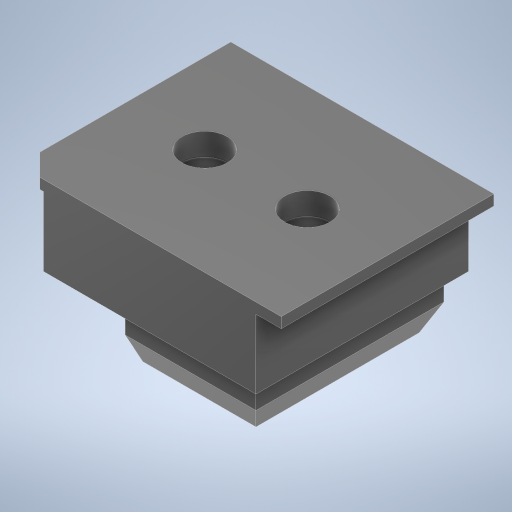
# Autodesk Inventor part: Header Larger Area
Saved by Autodesk Inventor 2024 (Build 280153000, 153)
## iProperties
Created: 2023-11-07
Part Number: Header Larger Area
Material: Acetal Resin, Black
Document SubType Name: Modeling
Designer: jamha
Density: 1.425 g/cm^3
Appearance: Smooth - Black
Author: jamha
Autodesk Inventor part; units mm, degrees
ref_plane "YZ Plane" through (0, 0, 0) normal (1, 0, 0) x (0, 1, 0)
ref_plane "XZ Plane" through (0, 0, 0) normal (0, 1, 0) x (-1, 0, 0)
ref_plane "XY Plane" through (0, 0, 0) normal (0, 0, 1) x (1, 0, 0)
ref_plane "Work Plane2" through (0, 3.81, 0) normal (0, 1, 0) x (1, 0, 0)
sketch "Sketch2" plane through (0, 3.81, 0) normal (0, 1, 0) x (1, 0, 0)
  line L0 (-29.21, 29.21) -> (1.27, 29.21)
  line L1 (1.27, -1.27) -> (-29.21, -1.27)
  line L2 (-29.21, -1.27) -> (-29.21, 29.21)
  line L3 (1.27, -1.27) -> (1.27, 29.21)
  line L4 (-4.8761, 25.94) -> (-25.94, 25.94) projected
  line L5 (-25.94, 25.94) -> (-25.94, 0) projected
  line L6 (-25.94, 0) -> (0, 0) projected
  line L7 (0, 0) -> (0, 21.0639) projected
  dimension "d3" = 30.48
  constraints: 8 end point, 3 equal length, 1 horizontal, 1 parallel, 1 vertical
  measures "d3" distance of L1.end L0.start
extrude "Extrusion2" add sketch "Sketch2" along normal blind 11.43
ref_plane "Work Plane1" through (0, -3.81, 0) normal (0, -1, 0) x (1, 0, 0)
ref_plane "Work Plane4" through (1.27, 3.81, -29.21) normal (0, 0, -1) x (-1, 0, 0)
sketch "Sketch6" plane through (1.27, 3.81, -29.21) normal (0, 0, -1) x (-1, 0, 0)
  line L0 (0, 11.43) -> (30.48, 11.43) projected
  line L1 (0, 11.43) -> (-7.239, 11.43)
  line L2 (-7.239, 11.43) -> (-7.239, 9.9183)
  line L3 (-7.239, 9.9183) -> (0, 9.9183)
  line L4 (0, 9.9183) -> (0, 11.43)
  line L5 (15.24, 11.43) -> (15.24, -7.62) construction
  line L6 (1.27, -7.62) -> (27.21, -7.62) construction
  line L7 (30.48, 11.43) -> (37.719, 11.43)
  line L8 (37.719, 11.43) -> (37.719, 9.9183)
  line L9 (37.719, 9.9183) -> (30.48, 9.9183)
  line L10 (30.48, 9.9183) -> (30.48, 11.43)
  point P0 (1.27, -3.81)
  dimension "d22" = 7.239
  constraints: 18 end point, 3 symmetric about line, 2 parallel, 1 horizontal, 1 midpoint, 1 perpendicular, 1 vertical, 2 other
  measures "d22" distance of L2.end L3.end
extrude "Extrusion6" add sketch "Sketch6" against normal up to surface (30.48 mm away)
ref_plane "Work Plane3" through (0, 15.24, 0) normal (0, 1, 0) x (1, 0, 0)
sketch "Sketch9" plane through (0, 15.24, 0) normal (0, 1, 0) x (1, 0, 0)
  line L0 (8.509, 29.21) -> (8.509, -1.27) construction
  line L1 (8.509, 13.97) -> (-36.449, 13.97) construction
  line L2 (-36.449, 29.21) -> (-36.449, -1.27) construction
  line L3 (-36.449, -1.27) -> (8.509, -1.27) construction
  line L4 (-13.97, -1.27) -> (-13.97, 29.21) construction
  line L5 (-36.449, 29.21) -> (8.509, 29.21) construction
  circle A0 centre (-21.336, 13.97) radius 3.2512
  circle A1 centre (-6.604, 13.97) radius 3.2512
  line L6 (-6.604, 13.97) -> (-21.336, 13.97) construction
  point P0 (0, 0)
  point P1 (-13.97, 13.97)
  point P2 (-13.97, 13.97)
  point P3 (-13.97, 13.97)
  point P4 (-13.97, 13.97)
  dimension "d25" = 14.732
  constraints: 6 end point, 6 midpoint, 3 coincident, 2 centre point, 1 horizontal
  measures "d25" distance of L6.end L6.start
extrude "Extrusion8" cut sketch "Sketch9" against normal blind 3.2258
ref_plane "Work Plane5" through (0, 15.24, 0) normal (0, 1, 0) x (1, 0, 0)
sketch "Sketch10" plane through (0, 15.24, 0) normal (0, 1, 0) x (1, 0, 0)
  line L0 (-29.21, -1.27) -> (-29.21, 29.21) projected
  line L1 (1.27, 29.21) -> (1.27, -1.27) projected
  line L2 (-36.449, 29.21) -> (-36.449, -1.27) projected
  line L3 (-36.449, 29.21) -> (8.509, 29.21) projected
  line L4 (-36.449, -1.27) -> (8.509, -1.27) projected
  line L5 (8.509, 29.21) -> (8.509, -1.27) projected
  line L6 (-29.21, 29.21) -> (-36.449, 29.21) projected
  line L7 (-29.21, 29.21) -> (-36.449, 29.21)
  line L8 (-32.8295, 29.21) -> (-32.8295, -1.27)
  line L9 (8.509, 29.21) -> (1.27, 29.21)
  line L10 (4.8895, 29.21) -> (4.8895, -1.27)
  line L11 (8.509, -1.27) -> (4.8895, -1.27)
  line L12 (8.509, 29.21) -> (8.509, -1.27) projected
  line L13 (8.509, 29.21) -> (8.509, -1.27)
  point P0 (0, 0)
  constraints: 12 end point, 4 collinear, 2 midpoint, 2 perpendicular, 2 point on line
extrude "Extrusion9" cut sketch "Sketch10" against normal blind 25.4 contours L4 L2 L3 L8 | L10 L3 L5 L4
sketch "Sketch18" plane through (0, 3.81, 0) normal (0, -1, 0) x (1, 0, 0)
  line L0 (1.27, 1.27) -> (1.27, -29.21) construction
  line L1 (1.27, -13.97) -> (-29.21, -13.97) construction
  line L2 (-29.21, -29.21) -> (-29.21, 1.27) construction
  line L3 (1.27, -29.21) -> (-29.21, -29.21) construction
  line L4 (-13.97, -29.21) -> (-13.97, 0) construction
  line L5 (0, -13.97) -> (-27.94, -13.97) construction
  line L6 (-13.97, 0) -> (-13.97, -27.94) construction
  line L7 (-13.97, -27.94) -> (-35.862, -27.94) construction
  line L8 (-20.7022, -26.44) -> (-37.4547, -26.44) construction
  line L9 (-27.44, -0.5) -> (-0.5, -0.5)
  line L10 (-0.5, -0.5) -> (-0.5, -27.44)
  line L11 (-0.5, -27.44) -> (-27.44, -27.44)
  line L12 (-27.44, -27.44) -> (-27.44, -0.5)
  line L13 (-27.44, -0.5) -> (-0.5, -27.44) construction
  line L14 (-0.5, -0.5) -> (-27.44, -27.44) construction
  line L15 (-27.44, -8.9624) -> (-18.9776, -0.5)
  point P0 (-13.97, -13.97)
  point P1 (-27.44, -20.8093)
  point P2 (-20.3093, -27.44)
  dimension "d66" = 1.27
  dimension "d72" = 26.94
  constraints: 26 end point, 7 midpoint, 5 point on line, 4 perpendicular, 2 horizontal, 2 parallel, 1 vertical
  measures "d66" distance between parallel lines of L3 L7
  measures "d72" distance of L10.end L11.end
extrude "Extrusion15" add sketch "Sketch18" along normal blind 7.62
sketch "Sketch19" plane through (0, -3.81, 0) normal (0, -1, 0) x (1, 0, 0)
  line L0 (-2.278, -2.278) -> (-2.278, -25.662) construction
  line L1 (-2.278, -13.97) -> (-25.662, -13.97) construction
  line L2 (-25.662, -25.662) -> (-25.662, -2.278) construction
  line L3 (-25.662, -2.278) -> (-2.278, -2.278) construction
  line L4 (-13.97, -2.278) -> (-13.97, -25.15) construction
  circle A0 centre (-13.97, -13.714) radius 2.0193
  point P0 (0, 0)
  point P1 (-25.412, -19.8229)
  dimension "d79" = 4.0386
  constraints: 4 end point, 3 midpoint, 1 centre point, 1 horizontal, 1 vertical, 2 other
  measures "d79" diameter of A0
extrude "Extrusion16" cut sketch "Sketch19" against normal blind 5.7404
sketch "Sketch21" plane through (0, -3.81, 0) normal (0, -1, 0) x (1, 0, 0)
  line L0 (-0.5, -0.5) -> (-27.44, -0.5) projected
  line L1 (-27.44, -0.5) -> (-27.44, -27.44) projected
  line L2 (-25.662, -2.278) -> (-27.44, -0.5) projected
  line L3 (-27.44, -8.7021) -> (-19.2379, -0.5)
  line L4 (-27.44, -8.7021) -> (-27.44, -0.5)
  point P0 (0, 0)
  constraints: 4 end point, 2 point on line, 1 collinear, 1 perpendicular
extrude "Extrusion18" cut sketch "Sketch21" against normal up to surface (7.62 mm away)
chamfer "Chamfer4" distance 1.778 angle 65 5 edges at (-9.869, -3.81, -0.5) (-23.339, -3.81, -4.601) (-27.44, -3.81, -18.071) (-13.97, -3.81, -27.44) (-0.5, -3.81, -13.97) measured on face at (-26.94, -3.81, -18.071) measured on face at (-13.97, -3.81, -26.94) measured on face at (-9.869, -3.81, -1) measured on face at (-1, -3.81, -13.97) measured on face at (-22.9854, -3.81, -4.9546)
sketch "Sketch22" plane through (0, 15.24, 0) normal (0, 1, 0) x (1, 0, 0)
  line L0 (-29.21, -1.27) -> (-32.8295, -1.27) projected
  line L1 (-32.8295, -1.27) -> (-29.972, 1.5875)
  line L2 (-32.8295, -1.27) -> (-28.7884, -1.27) construction
  line L3 (-29.6999, -1.27) -> (-32.8295, 1.8596)
  line L4 (-32.8295, -1.27) -> (-32.8295, 29.21) projected
  line L5 (-32.8295, 1.8596) -> (-32.8295, -1.27)
  point P0 (0, 0)
  dimension "d91" = 45
  constraints: 8 end point, 2 point on line, 1 collinear, 1 equal length, 1 horizontal, 1 perpendicular
  measures "d91" angle of L2 L1
extrude "Extrusion19" cut sketch "Sketch22" against normal up to surface (1.5117 mm away)
body "Solid1"
